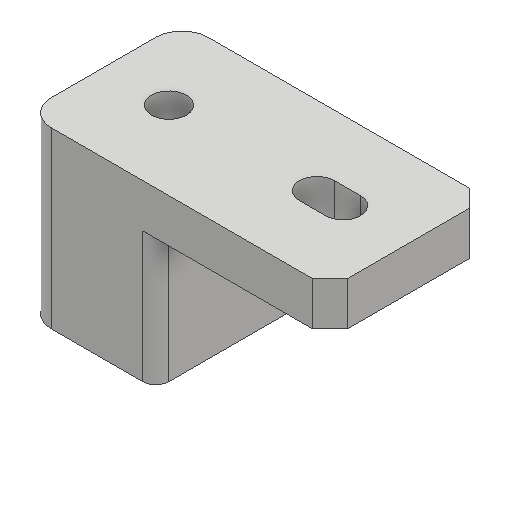
# Autodesk Inventor part: 3DP_ABS_X_End_Bearing_Mount
Saved by Autodesk Inventor 2026.1 (Build 301233000, 233)
## iProperties
Created: 2017-05-29
Part Number: 3DP_ABS_X_End_Bearing_Mount
Material: Ogólny
Document SubType Name: Modeling
Designer: Andrzej
Density: 1 g/cm^3
Appearance: Domyślna
Mass: 6.72858 g
Surface Area: 29.7095 cm^2
Volume: 6.72858 cm^3
Author: Andrzej
Autodesk Inventor part; units mm, degrees
ref_plane "YZ Plane" through (0, 0, 0) normal (1, 0, 0) x (0, 1, 0)
ref_plane "XZ Plane" through (0, 0, 0) normal (0, 1, 0) x (-1, 0, 0)
ref_plane "XY Plane" through (0, 0, 0) normal (0, 0, 1) x (1, 0, 0)
sketch "Szkic1" plane through (0, 0, 0) normal (0, 0, 1) x (1, 0, 0)
  line L0 (14.7767, -38.9659) -> (51.7767, -38.9659)
  line L1 (51.7767, -38.9659) -> (51.7767, -18.9659)
  line L2 (51.7767, -18.9659) -> (14.7767, -18.9659)
  line L3 (43.2767, -28.9659) -> (40.2767, -28.9659) construction
  line L4 (43.2767, -26.9659) -> (40.2767, -26.9659)
  line L5 (40.2767, -30.9659) -> (43.2767, -30.9659)
  arc A0 (43.2767, -30.9659) -> (43.2767, -26.9659) centre (43.2767, -28.9659) ccw
  arc A1 (40.2767, -26.9659) -> (40.2767, -30.9659) centre (40.2767, -28.9659) ccw
  line L6 (14.7767, -38.9659) -> (14.7767, -18.9659)
  line L7 (50.7767, -37.9659) -> (15.7767, -37.9659)
  line L8 (15.7767, -37.9659) -> (15.7767, -19.9659)
  line L9 (15.7767, -19.9659) -> (50.7767, -19.9659)
  line L10 (50.7767, -19.9659) -> (50.7767, -37.9659)
  line L11 (30.7767, -37.9659) -> (30.7767, -19.9659)
  point P0 (0, 0)
  point P1 (41.7767, -28.9659)
  dimension "d0" = 20
  dimension "d1" = 37
  dimension "d2" = 10
  dimension "d3" = 10
  dimension "d4" = 1.5
  dimension "d5" = 4
  dimension "d6" = 37
  dimension "d7" = 1
  dimension "d8" = 20
  constraints: 26 end point, 5 perpendicular, 4 point on circle, 4 tangent, 2 centre point, 2 horizontal, 2 point on line, 1 midpoint, 1 parallel, 3 other
  measures "d0" distance between parallel lines of L0 L2
  measures "d1" distance of L1.end L2.end
  measures "d2" distance from line of L1 point (41.777, -28.966)
  measures "d3" distance from line of L2 point (41.777, -28.966)
  measures "d4" distance of point (41.777, -28.966) L3.end
  measures "d5" diameter of A1
  measures "d6" distance of L0.start L1.start
  measures "d7" distance between parallel lines of L0 L7
  measures "d8" distance between parallel lines of L10 L11
extrude "Wyciągnięcie proste1" add sketch "Szkic1" along normal blind 5 contours L7 L11 L9 L10 | L7 L8 L9 L11
extrude "Wyciągnięcie proste2" add sketch "Szkic1" against normal blind 15 contours L7 L8 L9 L11
chamfer "Faza1" distance 2 angle 45 2 edges at (50.7767, -19.9659, 2.5) (50.7767, -37.9659, 2.5)
fillet "Zaokrąglenie1" radius 3 2 edges at (15.7767, -37.9659, -5) (15.7767, -19.9659, -5)
sketch "Szkic2" plane through (0, 0, -15) normal (0, 0, -1) x (-1, 0, 0)
  arc A0 (-15.7767, -22.9659) -> (-18.7767, -19.9659) centre (-18.7767, -22.9659) ccw projected
  line L0 (-18.7767, -19.9659) -> (-30.7767, -19.9659) projected
  line L1 (-30.7767, -19.9659) -> (-30.7767, -37.9659) projected
  line L2 (-30.7767, -37.9659) -> (-18.7767, -37.9659) projected
  arc A1 (-18.7767, -37.9659) -> (-15.7767, -34.9659) centre (-18.7767, -34.9659) ccw projected
  line L3 (-15.7767, -34.9659) -> (-15.7767, -22.9659) projected
  point P0 (0, 0)
  point P1 (-23.2767, -28.9659)
  dimension "d17" = 18
  dimension "d18" = 15
  dimension "d19" = 7.5
  dimension "d20" = 9
  measures "d17" distance between parallel lines of L0 L2
  measures "d18" distance between parallel lines of L1 L3
  measures "d19" distance from line of L3 point (-23.277, -28.966)
  measures "d20" distance from line of point (-23.277, -28.966) L2
hole "Otwór1" at (23.2767, -28.9659, -15) direction (0, 0, 1) diameter 4 end through all
fillet "Zaokrąglenie2" radius 1.5 2 edges at (30.7767, -37.9659, -7.5) (30.7767, -19.9659, -7.5)
equation "\"d6\" = d1"
equation "\"d19\" = 0.5 * d18"
equation "\"d20\" = 0.5 * d17"
